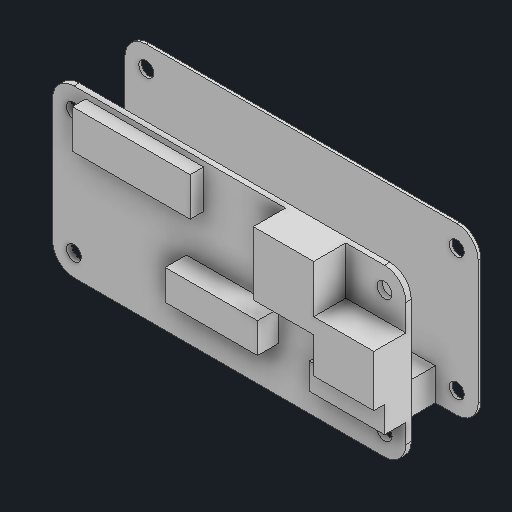
# Autodesk Inventor part: 라파+hat
Saved by Autodesk Inventor 2027.1 (Build 311270010, 270A)
## iProperties
Created: 2026-08-06
Part Number: 라파+hat
Material: 일반
Document SubType Name: Modeling
Designer: moieboy9999
Density: 4.25655 g/cm^3
Appearance: 기본값
Mass: 42 g
Surface Area: 102.708 cm^2
Volume: 9.86716 cm^3
Author: moieboy9999
Autodesk Inventor part; units mm, degrees
ref_plane "YZ Plane" through (0, 0, 0) normal (1, 0, 0) x (0, 1, 0)
ref_plane "XZ Plane" through (0, 0, 0) normal (0, 1, 0) x (-1, 0, 0)
ref_plane "XY Plane" through (0, 0, 0) normal (0, 0, 1) x (1, 0, 0)
sketch "스케치1" plane through (0, 0, 0) normal (0, 0, 1) x (1, 0, 0)
  circle A0 centre (0, 0) radius 1.4
  line L0 (0, 0) -> (58, 0)
  line L1 (58, 0) -> (58, -23)
  circle A1 centre (58, 0) radius 1.4
  circle A2 centre (0, -23) radius 1.4
  circle A3 centre (58, -23) radius 1.4
  line L2 (0, 0) -> (0, 4)
  line L3 (0, 4) -> (-4, 4)
  line L4 (0, 4) -> (58, 4)
  line L5 (62, 0) -> (62, -23)
  line L6 (58, -27) -> (0, -27)
  line L7 (-4, -23) -> (-4, 0)
  arc A4 (0, 4) -> (-4, 0) centre (0, 0) ccw
  arc A5 (62, 0) -> (58, 4) centre (58, 0) ccw
  arc A6 (58, -27) -> (62, -23) centre (58, -23) ccw
  arc A7 (-4, -23) -> (0, -27) centre (0, -23) ccw
  point P0 (62, -27)
  point P1 (62, 4)
  point P2 (-4, -27)
  dimension "d0" = 2.8
  dimension "d1" = 58
  dimension "d2" = 23
  dimension "d5" = 58
  dimension "d8" = 23
  dimension "d11" = 4
  dimension "d12" = 4
  dimension "d13" = 66
  dimension "d14" = 31
  dimension "d21" = 4
  constraints: 16 end point, 8 centre point, 8 point on circle, 8 point on line, 8 tangent, 3 equal radius, 3 horizontal, 3 perpendicular, 2 parallel, 2 vertical, 1 coincident, 6 other
  measures "d0" diameter of A0
  measures "d1" distance of L0.start L0.end
  measures "d2" distance of L0.end L1.end
  measures "d5" distance of L0.start A1.centre
  measures "d8" distance of L0.start A2.centre
  measures "d11" distance of L0.start L2.end
  measures "d12" distance of L2.end L3.end
  measures "d13" distance of point (62, -27) point (-4, -27)
  measures "d14" distance of point (62, 4) point (62, -27)
  measures "d21" radius of A4
extrude "돌출1" add sketch "스케치1" along normal blind 14
extrude "돌출2" cut sketch "스케치1" along normal blind 13
extrude "돌출3" add sketch "스케치1" along normal blind 1.5
sketch "스케치2" plane through (0, 0, 14) normal (0, 0, 1) x (1, 0, 0)
  line L0 (58, 4) -> (0, 4) projected
  line L1 (39.5003, 4) -> (50.7727, 4)
  line L2 (50.7727, 4) -> (50.7727, -7.8437)
  line L3 (50.7727, -7.8437) -> (39.5003, -7.8437)
  line L4 (39.5003, -7.8437) -> (39.5003, 4)
  line L5 (62, -23) -> (62, 0) projected
  line L6 (62, -4.9317) -> (50.7727, -4.9317)
  line L7 (50.7727, -4.9317) -> (50.7727, -14.5132)
  line L8 (50.7727, -14.5132) -> (62, -14.5132)
  line L9 (62, -14.5132) -> (62, -4.9317)
  line L10 (62, -14.5132) -> (47.9546, -14.5132)
  line L11 (47.9546, -14.5132) -> (47.9546, -19.3979)
  line L12 (47.9546, -19.3979) -> (62, -19.3979)
  line L13 (62, -19.3979) -> (62, -14.5132)
  line L14 (38.2792, -12.8223) -> (25.0341, -12.8223)
  line L15 (25.0341, -12.8223) -> (25.0341, -18.4585)
  line L16 (25.0341, -18.4585) -> (38.2792, -18.4585)
  line L17 (38.2792, -18.4585) -> (38.2792, -12.8223)
  point P0 (0, 0)
  point P1 (50.7727, -7.8437)
  constraints: 32 end point, 8 parallel, 4 horizontal, 4 perpendicular, 3 point on line
extrude "돌출4" add sketch "스케치2" along normal blind 6 contours L2 L3 L4 L0 | L6 L5 L8 L7 L2
extrude "돌출5" add sketch "스케치2" along normal blind 4 contours L8 L5 L12 L11 L10 | L17 L16 L15 L14
sketch "스케치3" plane through (0, 0, 1.5) normal (0, 0, 1) x (1, 0, 0)
  line L0 (0, -27) -> (58, -27) projected
  line L1 (29, -27) -> (4, -27)
  line L2 (4, -27) -> (54, -27)
  line L3 (54, -27) -> (54, -21)
  line L4 (54, -21) -> (4, -21)
  line L5 (4, -21) -> (4, -27)
  point P0 (0, 0)
  dimension "d26" = 25
  dimension "d27" = 50
  dimension "d28" = 6
  constraints: 10 end point, 2 parallel, 1 horizontal, 1 midpoint, 1 perpendicular, 1 point on line
  measures "d26" distance of L1.start L1.end
  measures "d27" distance of L4.end L3.end
  measures "d28" distance of L3.end L2.end
extrude "돌출6" add sketch "스케치3" along normal blind 12.25
extrude "돌출7" add sketch "스케치1" along normal blind 9.5
sketch "스케치4" plane through (0, 0, 0) normal (0, 0, -1) x (-1, 0, 0)
  line L0 (-4, -21) -> (-4, -27) projected
  line L1 (-4, -21) -> (-4, -27) projected
  line L2 (-54, -27) -> (-54, -21) projected
  line L3 (-54, -27) -> (-54, -21) projected
  line L4 (-54, -21) -> (-4, -21) projected
  line L5 (-54, -21) -> (-4, -21)
  line L6 (-4, -21) -> (-4, -27)
  line L7 (-4, -27) -> (-54, -27)
  line L8 (-54, -27) -> (-54, -21)
  point P0 (0, 0)
  constraints: 8 end point, 2 parallel, 1 horizontal, 1 perpendicular
extrude "돌출8" add sketch "스케치4" along normal blind 2
sketch "스케치5" plane through (0, 0, 14) normal (0, 0, 1) x (1, 0, 0)
  circle A0 centre (0, 0) radius 2.2
  line L0 (2.2, 0) -> (2.2, 3)
  line L1 (58, 4) -> (0, 4) projected
  line L2 (2.2, 3) -> (24.2, 3)
  line L3 (24.2, 3) -> (24.2, -4.2)
  line L4 (24.2, -4.2) -> (2.2, -4.2)
  line L5 (2.2, -4.2) -> (2.2, 3)
  dimension "d35" = 4.4
  dimension "d36" = 3
  dimension "d37" = 22
  dimension "d38" = 7.2
  constraints: 10 end point, 2 parallel, 2 perpendicular, 1 coincident, 1 horizontal, 1 horizontal alignment, 2 other
  measures "d36" distance of L0.start L0.end
  measures "d37" distance of L3.end L4.end
  measures "d38" distance of L2.end L3.end
extrude "돌출9" add sketch "스케치5" along normal blind 2.5 contours L0 L2 L3 L4 L5
move faces "이동1" translate (-4, 0, 0) faces at (25.0341, -14.7011, 15.3333)
move faces "이동2" translate (0, 0, -9) faces at (37.3333, -7.2234, 9.5)
